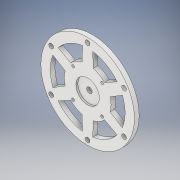
# Autodesk Inventor part: MC002
Saved by Autodesk Inventor 2017 SP1 (Build 210196100, 196)
## iProperties
Created: 2017-06-03
Part Number: MC002
Material: ABS Plastic
Document SubType Name: Modeling
Designer: Zach
Density: 1.06 g/cm^3
Appearance: CR White
Author: Zach
Autodesk Inventor part; units mm, degrees
ref_plane "YZ Plane" through (0, 0, 0) normal (1, 0, 0) x (0, 1, 0)
ref_plane "XZ Plane" through (0, 0, 0) normal (0, 1, 0) x (-1, 0, 0)
ref_plane "XY Plane" through (0, 0, 0) normal (0, 0, 1) x (1, 0, 0)
sketch "Sketch1" plane through (0, 0, 0) normal (0, 0, 1) x (1, 0, 0)
  circle A0 centre (0, 0) radius 50
  circle A1 centre (0, 0) radius 3
  circle A2 centre (0, 45) radius 2.5
  circle A3 centre (-38.9711, 22.5) radius 2.5
  circle A4 centre (-38.9711, -22.5) radius 2.5
  circle A5 centre (0, -45) radius 2.5
  circle A6 centre (38.9711, -22.5) radius 2.5
  circle A7 centre (38.9711, 22.5) radius 2.5
  dimension "d0" = 100
  dimension "d1" = 6
  dimension "d2" = 5
  dimension "d3" = 45
  dimension "d6" = 360
  constraints: 8 centre point, 2 coincident, 1 vertical alignment, 13 other
  measures "d0" diameter of A0
  measures "d1" diameter of A1
  measures "d2" diameter of A2
  measures "d3" distance of point (0, 0) A2.centre
extrude "Extrusion1" add sketch "Sketch1" along normal blind 5
sketch "Sketch2" plane through (0, 0, 5) normal (0, 0, 1) x (1, 0, 0)
  circle A0 centre (0, 0) radius 12.5
  dimension "d10" = 25
  constraints: 1 centre point, 1 coincident
  measures "d10" diameter of A0
extrude "Extrusion2" cut sketch "Sketch2" against normal blind 2
sketch "Sketch3" plane through (0, 0, 5) normal (0, 0, 1) x (1, 0, 0)
  circle A0 centre (0, 0) radius 3 projected
  circle A1 centre (0, 0) radius 25 construction
  circle A2 centre (0, 0) radius 40 construction
  line L0 (24, 7) -> (37.081, 15)
  line L1 (24, -7) -> (37.081, -15)
  line L2 (0, 0) -> (57.5693, 0) construction
  arc A3 (24, -7) -> (24, 7) centre (0, 0) ccw
  arc A4 (37.081, -15) -> (37.081, 15) centre (0, 0) ccw
  line L3 (5.9378, 24.2846) -> (5.5501, 39.6131)
  line L4 (18.0622, 17.2846) -> (31.5309, 24.6131)
  circle A5 centre (0, 0) radius 25 construction
  arc A6 (18.0622, 17.2846) -> (5.9378, 24.2846) centre (0, 0) ccw
  circle A7 centre (0, 0) radius 40 construction
  arc A8 (31.5309, 24.6131) -> (5.5501, 39.6131) centre (0, 0) ccw
  line L5 (-18.0622, 17.2846) -> (-31.5309, 24.6131)
  line L6 (-5.9378, 24.2846) -> (-5.5501, 39.6131)
  circle A9 centre (0, 0) radius 25 construction
  arc A10 (-5.9378, 24.2846) -> (-18.0622, 17.2846) centre (0, 0) ccw
  circle A11 centre (0, 0) radius 40 construction
  arc A12 (-5.5501, 39.6131) -> (-31.5309, 24.6131) centre (0, 0) ccw
  line L7 (-24, -7) -> (-37.081, -15)
  line L8 (-24, 7) -> (-37.081, 15)
  circle A13 centre (0, 0) radius 25 construction
  arc A14 (-24, 7) -> (-24, -7) centre (0, 0) ccw
  circle A15 centre (0, 0) radius 40 construction
  arc A16 (-37.081, 15) -> (-37.081, -15) centre (0, 0) ccw
  line L9 (-5.9378, -24.2846) -> (-5.5501, -39.6131)
  line L10 (-18.0622, -17.2846) -> (-31.5309, -24.6131)
  circle A17 centre (0, 0) radius 25 construction
  arc A18 (-18.0622, -17.2846) -> (-5.9378, -24.2846) centre (0, 0) ccw
  circle A19 centre (0, 0) radius 40 construction
  arc A20 (-31.5309, -24.6131) -> (-5.5501, -39.6131) centre (0, 0) ccw
  line L11 (18.0622, -17.2846) -> (31.5309, -24.6131)
  line L12 (5.9378, -24.2846) -> (5.5501, -39.6131)
  circle A21 centre (0, 0) radius 25 construction
  arc A22 (5.9378, -24.2846) -> (18.0622, -17.2846) centre (0, 0) ccw
  circle A23 centre (0, 0) radius 40 construction
  arc A24 (5.5501, -39.6131) -> (31.5309, -24.6131) centre (0, 0) ccw
  dimension "d13" = 50
  dimension "d14" = 80
  dimension "d15" = 15
  dimension "d16" = 7
  dimension "d19" = 360
  constraints: 48 point on circle, 26 end point, 24 centre point, 7 coincident, 7 concentric, 1 horizontal, 86 other
  measures "d13" diameter of A1
  measures "d14" diameter of A2
  measures "d15" vertical distance of point (0, 0) L0.end
  measures "d16" vertical distance of point (0, 0) L0.start
extrude "Extrusion3" cut sketch "Sketch3" against normal through all contours L0 A4 L1 A3 | L3 A8 L4 A6 | L5 A12 L6 A10 | L7 A16 L8 A14 | L9 A20 L10 A18 | L11 A24 L12 A22
sketch "Sketch5" plane through (0, 0, 5) normal (0, 0, 1) x (1, 0, 0)
  line L0 (-15.5, -15.5) -> (15.5, -15.5) construction
  line L1 (15.5, -15.5) -> (15.5, 15.5) construction
  line L2 (15.5, 15.5) -> (-15.5, 15.5) construction
  line L3 (-15.5, 15.5) -> (-15.5, -15.5) construction
  line L4 (-15.5, -15.5) -> (15.5, 15.5) construction
  line L5 (15.5, -15.5) -> (-15.5, 15.5) construction
  circle A0 centre (-15.5, 15.5) radius 1.5
  circle A1 centre (15.5, 15.5) radius 1.5
  circle A2 centre (15.5, -15.5) radius 1.5
  circle A3 centre (-15.5, -15.5) radius 1.5
  point P0 (0, 0)
  dimension "d23" = 31
  dimension "d24" = 31
  dimension "d25" = 3
  dimension "d26" = 3
  dimension "d27" = 3
  dimension "d28" = 3
  constraints: 12 end point, 4 centre point, 4 coincident, 2 midpoint, 2 parallel, 1 horizontal, 1 perpendicular
  measures "d23" distance of L2.end L1.end
  measures "d24" distance of L1.end L0.end
  measures "d25" diameter of A0
  measures "d26" diameter of A1
  measures "d27" diameter of A2
  measures "d28" diameter of A3
extrude "Extrusion4" cut sketch "Sketch5" against normal through all
equation "\"d29\" = d24"
body "Solid1"
